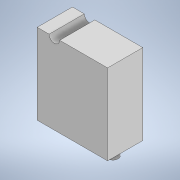
# Autodesk Inventor part: Support_2A
Saved by Autodesk Inventor 2021 (Build 250183000, 183)
## iProperties
Created: 2021-04-14
Part Number: Support_2A
Material: Generic
Document SubType Name: Modeling
Designer: Jawal
Density: 1 g/cm^3
Appearance: Default
Author: Jawal
Autodesk Inventor part; units mm, degrees
ref_plane "YZ Plane" through (0, 0, 0) normal (1, 0, 0) x (0, 1, 0)
ref_plane "XZ Plane" through (0, 0, 0) normal (0, 1, 0) x (-1, 0, 0)
ref_plane "XY Plane" through (0, 0, 0) normal (0, 0, 1) x (1, 0, 0)
sketch "Sketch1" plane through (0, 0, 0) normal (1, 0, 0) x (0, 1, 0)
  line L0 (11.4385, 5) -> (-11.4385, 5)
  line L1 (-11.4385, 5) -> (-11.4385, -5)
  line L2 (-11.4385, -5) -> (11.4385, -5)
  line L3 (11.4385, -5) -> (11.4385, 5)
  point P0 (0, 0)
  dimension "d0" = 22.877
  dimension "d1" = 11.4385
  dimension "d3" = 10
  dimension "d4" = 5
  constraints: 8 end point, 2 parallel, 1 horizontal, 1 perpendicular
  measures "d0" distance of L1.end L2.end
  measures "d1" distance from line of point (0, 0) L3
  measures "d3" distance of L2.end L0.start
  measures "d4" distance from line of point (0, 0) L0
extrude "Extrusion1" add sketch "Sketch1" along normal blind 20
sketch "Sketch2" plane through (0, -11.4385, -5) normal (0, -1, 0) x (1, 0, 0)
  circle A0 centre (16.5, 5) radius 1.5
  line L0 (20, 10) -> (20, 0) projected
  point P0 (0, 5)
  dimension "d7" = 3
  dimension "d8" = 3.5
  constraints: 1 centre point
  measures "d7" diameter of A0
  measures "d8" distance from line of L0 A0.centre
extrude "Extrusion2" add sketch "Sketch2" along normal blind 3
sketch "Sketch3" plane through (0, -11.4385, 5) normal (0, 0, 1) x (1, 0, 0)
  line L0 (0, 22.877) -> (20, 22.877) projected
  arc A0 (3.387, 22.877) -> (6.387, 22.877) centre (4.887, 22.877) ccw
  line L1 (0, 22.877) -> (0, 0) projected
  line L2 (3.387, 22.877) -> (6.387, 22.877)
  line L3 (0, 22.877) -> (20, 22.877) projected
  point P0 (0, 11.4385)
  dimension "d11" = 3
  dimension "d12" = 4.887
  constraints: 3 point on line, 2 end point, 2 point on circle, 1 centre point, 1 collinear
  measures "d11" diameter of A0
  measures "d12" distance from line of L1 A0.centre
extrude "Extrusion3" cut sketch "Sketch3" against normal through all
equation "\"d1\" = 0.5 * d0"
equation "\"d4\" = 0.5 * d3"
body "Solid1"
